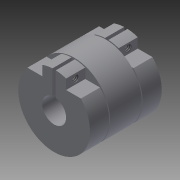
# Autodesk Inventor part: Flexible Shaft Coupler 6208K411
Saved by Autodesk Inventor 2013 (Build 170138000, 138)
## iProperties
Created: 2013-06-25
Part Number: Flexible Shaft Coupler 6208K411
Material: Generic
Document SubType Name: Modeling
Designer: mvarma
Density: 1 g/cm^3
Author: mvarma
Autodesk Inventor part; units mm, degrees
ref_plane "YZ Plane" through (0, 0, 0) normal (1, 0, 0) x (0, 1, 0)
ref_plane "XZ Plane" through (0, 0, 0) normal (0, 1, 0) x (-1, 0, 0)
ref_plane "XY Plane" through (0, 0, 0) normal (0, 0, 1) x (1, 0, 0)
sketch "Sketch1" plane through (0, 0, 0) normal (0, 0, 1) x (1, 0, 0)
  circle A0 centre (0, 0) radius 9.525
  circle A1 centre (0, 0) radius 3.175
  line L0 (0, 0) -> (-0.4464, 0)
  line L1 (-0.4464, 0) -> (-0.4464, 9.5145)
  line L2 (0, 0) -> (0.4464, 0)
  line L3 (0.4464, 0) -> (0.4464, 9.5145)
  line L4 (0, 0) -> (0, 9.525)
  line L5 (-7.0995, 6.35) -> (-3.175, 6.35)
  line L6 (-3.175, 6.35) -> (-3.175, 8.9803)
  line L7 (3.175, 8.9803) -> (3.175, 6.35)
  line L8 (3.175, 6.35) -> (7.0995, 6.35)
  dimension "d0" = 19.05
  dimension "d1" = 6.35
  dimension "d4" = 3.175
  dimension "d5" = 0.4464
  dimension "d6" = 3.175
  dimension "d7" = 3.175
  constraints: 18 end point, 6 perpendicular, 2 coincident, 2 parallel, 1 centre point, 1 horizontal, 11 other
  measures "d1" diameter of A1
  measures "d4" distance between parallel lines of L6 L4
  measures "d5" distance between parallel lines of L1 L4
  measures "d6" distance from line of L4.end L5
  measures "d7" distance from line of L4.end L8
extrude "Extrusion1" add sketch "Sketch1" along normal blind 19.05
extrude "Extrusion2" cut sketch "Sketch1" along normal blind 5.334 contours L8 L7 A0 | A0 L6 L5 | L3 A1 L4 A0 | A0 L4 A1 L1 | L3 L2 L4 A1 | A1 L1 L0 L2 L3 | A1 L4 L0 L1
sketch "Sketch2" plane through (0, 0, 5.334) normal (0, 0, -1) x (-1, 0, 0)
  line L0 (-3.175, 8.9803) -> (-3.175, 6.35) projected
  arc A0 (-3.175, 8.9803) -> (-7.0995, 6.35) centre (0, 0) ccw projected
  line L1 (-3.175, 6.35) -> (-7.0995, 6.35) projected
  circle A1 centre (0, 0) radius 9.525
  line L2 (-7.0995, -6.35) -> (7.0995, -6.35)
  dimension "d10" = 6.35
  constraints: 3 point on circle, 2 end point, 1 centre point, 1 coincident, 1 parallel
  measures "d10" distance from line of A1.centre L2
extrude "Extrusion3" cut sketch "Sketch2" along normal blind 0.254 contours A1 L2 L1 L0
ref_plane "Work Plane1" through (0, 0, 9.525) normal (0, 0, -1) x (-1, 0, 0)
sketch "Sketch3" plane through (3.175, 6.35, 0) normal (1, 0, 0) x (0, 0, -1)
  line L0 (0, 0) -> (-5.08, 0) projected
  line L1 (0, 2.6303) -> (0, 0) projected
  point P0 (0, -6.35)
  point P1 (-2.54, 1.3151)
  dimension "d14" = 2.54
  dimension "d15" = 1.3151
  measures "d14" distance from line of point (-2.54, 1.315) L1
  measures "d15" distance from line of point (-2.54, 1.315) L0
hole "Hole1" at (3.175, 7.6651, 2.54) direction (-1, 0, 0) diameter 1.7018 depth 25.4 tip angle 118
mirror "Mirror1" about plane through (0, 0, 9.525) normal (0, 0, -1) of "Extrusion2", "Extrusion3", "Hole1"
equation "\"d7\" = d6"
body "Solid1"
